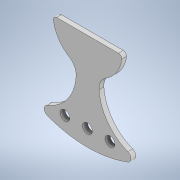
# Autodesk Inventor part: 中間ユニット外
Saved by Autodesk Inventor 2022.2 (Build 262287000, 287)
## iProperties
Created: 2022-01-03
Part Number: 中間ユニット外
Material: Generic
Document SubType Name: Modeling
Designer: acps
Density: 1 g/cm^3
Appearance: Default
Author: acps
Autodesk Inventor part; units mm, degrees
ref_plane "YZ Plane" through (0, 0, 0) normal (1, 0, 0) x (0, 1, 0)
ref_plane "XZ Plane" through (0, 0, 0) normal (0, 1, 0) x (-1, 0, 0)
ref_plane "XY Plane" through (0, 0, 0) normal (0, 0, 1) x (1, 0, 0)
sketch "Sketch1" plane through (0, 0, 0) normal (0, 0, 1) x (1, 0, 0)
  circle A0 centre (16.2, 5) radius 9.025
  arc A1 (15.9625, 14.0219) -> (35.7029, 29.6112) centre (15.41, 35.0146) ccw
  arc A2 (8.6866, 0) -> (52.5133, -3.5421) centre (31.9968, 15.5125) ccw
  circle A3 centre (16.2, 5) radius 6.025
  arc A4 (70.0205, 42.4797) -> (35.7029, 29.6112) centre (57.4454, 23.8218) ccw
  circle A5 centre (14, -20) radius 3
  circle A6 centre (0, -20) radius 3
  circle A7 centre (-14, -20) radius 3
  line L0 (16.2, 5) -> (136.0469, 5) construction
  line L1 (16.2, 5) -> (120.1794, 65.0325) construction
  line L2 (16.2, 5) -> (136.265, 5) construction
  line L3 (16.2, 5) -> (121.2083, -55.6266) construction
  line L4 (16.2, 5) -> (137.4531, 5) construction
  arc A8 (11.4834, 12.6944) -> (20.7844, 36.0654) centre (0.5085, 30.5984) ccw construction
  arc A9 (7.1931, 4.4289) -> (43.377, -20.5519) centre (35.1365, 6.208) ccw construction
  arc A10 (11.4312, 12.7797) -> (21.4, 30) centre (0.5085, 30.5984) ccw
  line L5 (21.4, 30) -> (0, 30)
  arc A11 (7.0935, 4.4191) -> (25, -20) centre (35.1365, 6.208) ccw
  arc A12 (11.4312, 12.7797) -> (7.0935, 4.4191) centre (16.2, 5) ccw
  line L6 (0, 30) -> (0, -48.3313) construction
  line L7 (-21.4, 30) -> (0, 30)
  arc A13 (-21.4, 30) -> (-11.4312, 12.7797) centre (-0.5085, 30.5984) ccw
  arc A14 (-7.0935, 4.4191) -> (-11.4312, 12.7797) centre (-16.2, 5) ccw
  arc A15 (-25, -20) -> (-7.0935, 4.4191) centre (-35.1365, 6.208) ccw
  line L8 (-36.0984, -20) -> (40.4938, -20)
  circle A16 centre (23.9178, -22.798) radius 3
  circle A17 centre (-23.9178, -22.798) radius 3
  arc A18 (-24.9888, -25.6003) -> (24.9888, -25.6003) centre (0, 39.7874) ccw
  line L9 (-31.4755, -75) -> (165.3406, -75) construction
  point P0 (0, 0)
  point P1 (25.2806, -20)
  point P2 (-25.2806, -20)
  point P3 (-20.9441, -22.4019)
  point P4 (28.425, 18.534)
  dimension "d0" = 6
  dimension "d1" = 6
  dimension "d2" = 6
  dimension "d3" = 30
  dimension "d4" = 30
  dimension "d5" = 0.1
  dimension "d6" = 0.1
  dimension "d7" = 20.9
  dimension "d8" = 9.125
  dimension "d9" = 30
  dimension "d10" = 20
  dimension "d11" = 21.4
  dimension "d12" = 28
  dimension "d13" = 6
  dimension "d14" = 6
  dimension "d15" = 70
  dimension "d16" = 14
  dimension "d17" = 14
  dimension "d18" = 25
  dimension "d19" = 75
  constraints: 31 point on circle, 20 end point, 19 centre point, 7 horizontal, 7 point on line, 7 symmetric about line, 6 tangent, 2 equal length, 2 vertical, 11 other
  measures "d0" diameter of A5
  measures "d1" diameter of A6
  measures "d2" diameter of A7
  measures "d3" angle of L2 L1
  measures "d4" angle of L3 L4
  measures "d5" radial gap between concentric circles of A8 A10
  measures "d6" radial gap between concentric circles of A9 A11
  measures "d7" radius of A10
  measures "d8" radius of A12
  measures "d9" distance from line of point (0, 0) L7
  measures "d10" distance from line of L8 point (0, 0)
  measures "d11" distance of L5.start L5.end
  measures "d12" radius of A9
  measures "d13" diameter of A16
  measures "d14" diameter of A17
  measures "d15" radius of A18
  measures "d16" distance of A5.centre A6.centre
  measures "d17" distance of A7.centre A6.centre
  measures "d18" distance of A11.end A6.centre
  measures "d19" distance from line of L9 point (0, 0)
extrude "Extrusion1" add sketch "Sketch1" along normal blind 3 contours L8 A16 A18 A17 A7 A6 A5 | A5 L8 A6 A7 A17 A15 A14 A13 L7 L5 A10 A12 A11 A16 | A16 L8 | L8 A16 | A17 L8 | A17 L8
fillet "Fillet1" radius 2 2 edges at (21.4, 30, 1.5) (-21.4, 30, 1.5)
body "Solid1"
